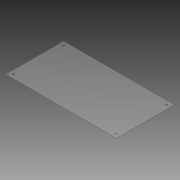
# Autodesk Inventor part: Polycarbonate Facia
Saved by Autodesk Inventor 2015 (Build 190159000, 159)
## iProperties
Created: 2014-08-06
Part Number: Polycarbonate Facia
Material: Polycarbonate, Clear
Document SubType Name: Modeling
Designer: simon
Density: 1.2 g/cm^3
Appearance: Polycarbonate - Clear
Author: simon
Autodesk Inventor part; units mm, degrees
ref_plane "YZ Plane" through (0, 0, 0) normal (1, 0, 0) x (0, 1, 0)
ref_plane "XZ Plane" through (0, 0, 0) normal (0, 1, 0) x (-1, 0, 0)
ref_plane "XY Plane" through (0, 0, 0) normal (0, 0, 1) x (1, 0, 0)
sketch "Sketch1" plane through (0, 0, 0) normal (0, 0, 1) x (1, 0, 0)
  line L0 (0, 0) -> (145.9, 0)
  line L1 (145.9, 0) -> (145.9, 75.9)
  line L2 (145.9, 75.9) -> (0, 75.9)
  line L3 (0, 75.9) -> (0, 0)
  dimension "d0" = 145.9
  dimension "d1" = 75.9
  constraints: 8 end point, 2 parallel, 1 horizontal, 1 perpendicular
  measures "d0" distance of L2.end L1.end
  measures "d1" distance of L1.end L0.end
extrude "Extrusion1" add sketch "Sketch1" along normal blind 1
sketch "Sketch2" plane through (0, 0, 1) normal (0, 0, 1) x (1, 0, 0)
  line L0 (145.9, 75.9) -> (0, 75.9) construction
  line L1 (0, 75.9) -> (0, 0) construction
  line L2 (0, 0) -> (145.9, 0) construction
  line L3 (145.9, 0) -> (145.9, 75.9) construction
  line L4 (145.9, 75.9) -> (0, 75.9) construction
  line L5 (0, 75.9) -> (0, 0) construction
  line L6 (141.05, 4.85) -> (4.85, 4.85) construction
  line L7 (4.85, 4.85) -> (4.85, 71.05) construction
  line L8 (4.85, 71.05) -> (141.05, 71.05) construction
  line L9 (141.05, 71.05) -> (141.05, 4.85) construction
  dimension "d4" = 4.85
  constraints: 8 end point, 4 coincident, 3 other
  measures "d4" distance between parallel lines of L2 L6
hole "Hole1" at (4.85, 71.05, 1) at (4.85, 4.85, 1) at (141.05, 4.85, 1) at (141.05, 71.05, 1) direction (0, 0, -1) diameter 3 end through all
sketch "Sketch3" plane through (0, 0, 0) normal (0, 0, -1) x (-1, 0, 0)
  circle A0 centre (-141.05, 4.85) radius 1.5 construction
  circle A1 centre (-4.85, 71.05) radius 1.5 construction
  circle A2 centre (-4.85, 4.85) radius 1.5 construction
  circle A3 centre (-141.05, 71.05) radius 1.5 construction
  line L0 (0, 0) -> (-145.9, 0) construction
  line L1 (0, 75.9) -> (0, 0) construction
  line L2 (-145.9, 75.9) -> (0, 75.9) construction
  line L3 (-145.9, 0) -> (-145.9, 75.9) construction
  line L4 (-68.15, 0) -> (-68.15, 75.9) construction
  line L5 (0, 9.45) -> (-68.15, 9.45) construction
  line L6 (0, 28.45) -> (-68.15, 28.45) construction
  line L7 (0, 47.45) -> (-68.15, 47.45) construction
  line L8 (0, 66.45) -> (-68.15, 66.45) construction
  circle A4 centre (-68.15, 9.45) radius 7.5
  circle A5 centre (-68.15, 28.45) radius 7.5
  circle A6 centre (-68.15, 47.45) radius 7.5
  circle A7 centre (-68.15, 66.45) radius 7.5
  dimension "d20" = 68.15
  dimension "d21" = 9.45
  dimension "d23" = 19
  dimension "d24" = 19
  dimension "d25" = 19
  dimension "d26" = 15
  dimension "d27" = 15
  dimension "d28" = 15
  dimension "d29" = 15
  constraints: 10 end point, 10 point on line, 4 centre point, 4 coincident, 4 perpendicular, 1 horizontal
  measures "d20" distance between parallel lines of L1 L4
  measures "d21" distance between parallel lines of L5 L0
  measures "d23" distance between parallel lines of L6 L5
  measures "d24" distance between parallel lines of L7 L6
  measures "d25" distance between parallel lines of L8 L7
  measures "d26" diameter of A4
  measures "d27" diameter of A5
  measures "d28" diameter of A6
  measures "d29" diameter of A7
extrude "Extrusion2" cut sketch "Sketch3" against normal blind 0.001
body "Solid1"
